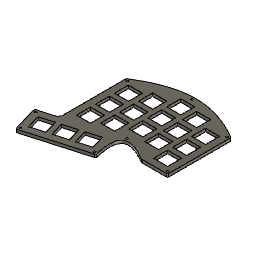
mrkabuda_switch_plate_19 v3 (Autodesk Fusion 360 design; units mm, degrees)
Autodesk Fusion 360 part; units mm, degrees
sketch "Sketch1" plane through (0, 0, 0) normal (0, 0, 1) x (1, 0, 0)
  line L0 (-65.1137, -18.4026) -> (-58.0679, -42.9099)
  line L1 (-56.8305, -43.5946) -> (3.7699, -26.1721)
  line L2 (32.056, -7.0618) -> (56.5101, -7.0618)
  line L3 (57.5101, -6.0618) -> (57.5101, 55.7146)
  line L4 (-45.9899, 54.3854) -> (-45.9899, -8.099)
  line L5 (-49.6083, -12.9043) -> (-64.4289, -17.1652)
  line L6 (-39.2399, 50.5) -> (-25.2399, 50.5)
  line L7 (-25.2399, 50.5) -> (-25.2399, 36.5)
  line L8 (-25.2399, 36.5) -> (-39.2399, 36.5)
  line L9 (-39.2399, 36.5) -> (-39.2399, 50.5)
  line L10 (-39.2399, 31.5) -> (-25.2399, 31.5)
  line L11 (-25.2399, 31.5) -> (-25.2399, 17.5)
  line L12 (-25.2399, 17.5) -> (-39.2399, 17.5)
  line L13 (-39.2399, 17.5) -> (-39.2399, 31.5)
  line L14 (-39.2399, 12.5) -> (-25.2399, 12.5)
  line L15 (-25.2399, 12.5) -> (-25.2399, -1.5)
  line L16 (-25.2399, -1.5) -> (-39.2399, -1.5)
  line L17 (-39.2399, -1.5) -> (-39.2399, 12.5)
  line L18 (-6.2399, 17.7863) -> (-6.2399, 3.7863)
  line L19 (-20.2399, 17.7863) -> (-6.2399, 17.7863)
  line L20 (-6.2399, 3.7863) -> (-20.2399, 3.7863)
  line L21 (-6.2399, 36.7863) -> (-6.2399, 22.7863)
  line L22 (-6.2399, 22.7863) -> (-20.2399, 22.7863)
  line L23 (-6.2399, 55.7863) -> (-6.2399, 41.7863)
  line L24 (-20.2399, 41.7863) -> (-20.2399, 55.7863)
  line L25 (-20.2399, 22.7863) -> (-20.2399, 36.7863)
  line L26 (-20.2399, 36.7863) -> (-6.2399, 36.7863)
  line L27 (-6.2399, 41.7863) -> (-20.2399, 41.7863)
  line L28 (-20.2399, 55.7863) -> (-6.2399, 55.7863)
  line L29 (-20.2399, 3.7863) -> (-20.2399, 17.7863)
  line L30 (12.7601, 26.8291) -> (12.7601, 12.8291)
  line L31 (-1.2399, 26.8291) -> (12.7601, 26.8291)
  line L32 (12.7601, 12.8291) -> (-1.2399, 12.8291)
  line L33 (12.7601, 45.8291) -> (12.7601, 31.8291)
  line L34 (12.7601, 31.8291) -> (-1.2399, 31.8291)
  line L35 (12.7601, 64.8291) -> (12.7601, 50.8291)
  line L36 (-1.2399, 50.8291) -> (-1.2399, 64.8291)
  line L37 (-1.2399, 31.8291) -> (-1.2399, 45.8291)
  line L38 (-1.2399, 45.8291) -> (12.7601, 45.8291)
  line L39 (12.7601, 50.8291) -> (-1.2399, 50.8291)
  line L40 (-1.2399, 64.8291) -> (12.7601, 64.8291)
  line L41 (-1.2399, 12.8291) -> (-1.2399, 26.8291)
  line L42 (31.7601, 23.77) -> (31.7601, 9.77)
  line L43 (17.7601, 23.77) -> (31.7601, 23.77)
  line L44 (31.7601, 9.77) -> (17.7601, 9.77)
  line L45 (31.7601, 42.77) -> (31.7601, 28.77)
  line L46 (31.7601, 28.77) -> (17.7601, 28.77)
  line L47 (31.7601, 61.77) -> (31.7601, 47.77)
  line L48 (17.7601, 47.77) -> (17.7601, 61.77)
  line L49 (17.7601, 28.77) -> (17.7601, 42.77)
  line L50 (17.7601, 42.77) -> (31.7601, 42.77)
  line L51 (31.7601, 47.77) -> (17.7601, 47.77)
  line L52 (17.7601, 61.77) -> (31.7601, 61.77)
  line L53 (17.7601, 9.77) -> (17.7601, 23.77)
  line L54 (50.7601, 13.6882) -> (50.7601, -0.3118)
  line L55 (36.7601, 13.6882) -> (50.7601, 13.6882)
  line L56 (50.7601, -0.3118) -> (36.7601, -0.3118)
  line L57 (50.7601, 32.6882) -> (50.7601, 18.6882)
  line L58 (50.7601, 18.6882) -> (36.7601, 18.6882)
  line L59 (50.7601, 51.6882) -> (50.7601, 37.6882)
  line L60 (36.7601, 37.6882) -> (36.7601, 51.6882)
  line L61 (36.7601, 18.6882) -> (36.7601, 32.6882)
  line L62 (36.7601, 32.6882) -> (50.7601, 32.6882)
  line L63 (50.7601, 37.6882) -> (36.7601, 37.6882)
  line L64 (36.7601, 51.6882) -> (50.7601, 51.6882)
  line L65 (36.7601, -0.3118) -> (36.7601, 13.6882)
  line L66 (-57.0377, -22.0637) -> (-53.1694, -35.5187)
  line L67 (-53.1694, -35.5187) -> (-39.7144, -31.6504)
  line L68 (-39.7144, -31.6504) -> (-43.5827, -18.1954)
  line L69 (-43.5827, -18.1954) -> (-57.0377, -22.0637)
  line L70 (-38.7774, -16.8139) -> (-34.9091, -30.2689)
  line L71 (-34.9091, -30.2689) -> (-21.4541, -26.4006)
  line L72 (-21.4541, -26.4006) -> (-25.3224, -12.9456)
  line L73 (-25.3224, -12.9456) -> (-38.7774, -16.8139)
  line L74 (-7.0621, -7.6958) -> (-20.517, -11.5641)
  line L75 (-3.1938, -21.1508) -> (-7.0621, -7.6958)
  line L76 (-20.517, -11.5641) -> (-16.6488, -25.019)
  line L77 (-16.6488, -25.019) -> (-3.1938, -21.1508)
  arc A0 (30.9232, -6.9303) -> (32.056, -7.0618) centre (32.0625, -2.0618) ccw
  arc A1 (56.5101, -7.0618) -> (57.5101, -6.0618) centre (56.5101, -6.0618) ccw
  arc A2 (-49.6083, -12.9043) -> (-45.9899, -8.099) centre (-50.9899, -8.099) ccw
  arc A3 (-64.4289, -17.1652) -> (-65.1137, -18.4026) centre (-64.1526, -18.1263) ccw
  arc A4 (-58.0679, -42.9099) -> (-56.8305, -43.5946) centre (-57.1068, -42.6336) ccw
  spline S0 degree 5 poles (4.4658, -24.9769) (4.0861, -23.4005) (3.405, -20.3536) (2.618, -16.1015) (2.0468, -11.0788) (2.1888, -5.9515) (3.2681, -2.0775) (5.3643, 0.4418) (8.517, 1.5538) (12.6793, 1.3152) (17.7712, -0.1754) (22.5239, -2.2909) (26.4446, -4.3657) (29.214, -5.9628) (30.6376, -6.8147) knots 0 0 0 0 0 0 0.1 0.2 0.3 0.4 0.5 0.6 0.7 0.8 0.9 1 1 1 1 1 1
  spline S1 degree 5 poles (-45.5293, 55.2274) (-43.5173, 56.5166) (-39.4897, 58.9843) (-33.4382, 62.3543) (-25.3488, 66.1735) (-15.1999, 69.7485) (-5.0108, 72.0184) (5.2219, 72.8785) (15.4996, 72.2738) (25.8202, 70.2648) (36.1806, 66.9583) (44.4983, 63.3605) (50.7521, 60.1603) (54.9281, 57.8074) (57.0178, 56.5761) knots 0 0 0 0 0 0 0.1 0.2 0.3 0.4 0.5 0.6 0.7 0.8 0.9 1 1 1 1 1 1
  arc A5 (57.5101, 55.7146) -> (57.0178, 56.5761) centre (56.5101, 55.7146) ccw
  arc A6 (-45.5293, 55.2274) -> (-45.9899, 54.3854) centre (-44.9899, 54.3854) ccw
  arc A7 (3.7699, -26.1721) -> (4.4658, -24.9769) centre (3.4936, -25.2111) ccw
  arc A8 (30.6376, -6.8147) -> (30.9232, -6.9303) centre (31.1511, -5.9566) ccw
  line L78 (6.3992, -33.0044) -> (2.5325, -16.9495)
  circle A9 centre (-43.4899, 53.565) radius 1.05
  line L79 (-55.3639, 48.9264) -> (-35.6948, 61.5285)
  circle A10 centre (4.9998, 70.0097) radius 1.05
  line L80 (-4.8791, 72.3551) -> (14.8791, 72.6649)
  circle A11 centre (55.0101, 54.8574) radius 1.05
  line L81 (46.894, 62.5413) -> (67.1415, 50.611)
  circle A12 centre (55.0101, -4.5618) radius 1.05
  circle A13 centre (6.2551, 3.6516) radius 1.05
  circle A14 centre (1.6991, -24.1662) radius 1.05
  line L82 (3.2764, -1.6283) -> (7.7236, 1.6283)
  circle A15 centre (-56.0797, -40.7775) radius 1.05
  circle A16 centre (-62.2965, -19.1534) radius 1.05
  point P0 (-57.7916, -43.8709)
  point P1 (5.5, 0)
  point P2 (5, 72.51)
  dimension "d1" = 27.5
  dimension "d2" = 14
  dimension "d3" = 14
  dimension "d4" = 14
  dimension "d5" = 14
  dimension "d6" = 14
  dimension "d7" = 14
  dimension "d18" = 14
  dimension "d19" = 14
  dimension "d20" = 14
  dimension "d21" = 14
  dimension "d22" = 14
  dimension "d23" = 14
  dimension "d26" = 14
  dimension "d27" = 14
  dimension "d28" = 14
  dimension "d29" = 14
  dimension "d30" = 14
  dimension "d31" = 14
  dimension "d34" = 14
  dimension "d35" = 14
  dimension "d36" = 14
  dimension "d37" = 14
  dimension "d38" = 14
  dimension "d39" = 14
  dimension "d42" = 14
  dimension "d43" = 14
  dimension "d44" = 14
  dimension "d45" = 14
  dimension "d46" = 14
  dimension "d47" = 14
  dimension "d48" = 5
  dimension "d50" = 5
  dimension "d51" = 5
  dimension "d52" = 5
  dimension "d53" = 5
  dimension "d54" = 5
  dimension "d55" = 5
  dimension "d59" = 5
  dimension "d66" = 14
  dimension "d67" = 14
  dimension "d70" = 14
  dimension "d71" = 14
  dimension "d73" = 14
  dimension "d74" = 14
  dimension "d77" = 6.75
  dimension "d80" = 1
  dimension "d83" = 5
  dimension "d85" = 1
  dimension "d86" = 1
  dimension "d135" = 6.75
  dimension "d139" = 1
  dimension "d140" = 1
  dimension "d141" = 1
  dimension "d142" = 1
  dimension "d175" = 2.1
  dimension "d176" = 2.5
  dimension "d177" = 2.5
  dimension "d178" = 2.1
  dimension "d179" = 2.5
  dimension "d180" = 2.1
  dimension "d181" = 2.5
  dimension "d182" = 2.5
  dimension "d183" = 2.1
  dimension "d184" = 2.5
  dimension "d185" = 2.5
  dimension "d186" = 2.1
  dimension "d187" = 2.1
  dimension "d188" = 2.5
  dimension "d189" = 2.5
  dimension "d190" = 2.5
  dimension "d191" = 2.1
  dimension "d192" = 2.5
  dimension "d193" = 2.5
  dimension "d194" = 2.1
  dimension "d195" = 2.5
  dimension "d196" = 2.5
  dimension "d197" = 6.75
  dimension "d198" = 6.75
  dimension "d199" = 6.75
  dimension "d201" = 5
  dimension "d202" = 6.75
  dimension "d203" = 6.75
  dimension "d204" = 5
  dimension "d205" = 5
  dimension "d206" = 5
  dimension "d207" = 5
  dimension "d208" = 5
  dimension "d209" = 5
  dimension "d210" = 5
  dimension "d211" = 5
  dimension "d212" = 5
  dimension "d214" = 5
  dimension "d215" = 5
  constraint horizontal L2
  constraint perpendicular L2 L3
  constraint perpendicular L2 L4
  constraint horizontal L6
  constraint vertical L7
  constraint horizontal L8
  constraint vertical L9
  constraint horizontal L10
  constraint vertical L11
  constraint horizontal L12
  constraint vertical L13
  constraint horizontal L14
  constraint vertical L15
  constraint horizontal L16
  constraint vertical L17
  constraint horizontal L28
  constraint vertical L23
  constraint horizontal L27
  constraint vertical L24
  constraint horizontal L26
  constraint vertical L21
  constraint horizontal L22
  constraint vertical L25
  constraint horizontal L19
  constraint vertical L18
  constraint horizontal L20
  constraint vertical L29
  constraint horizontal L40
  constraint vertical L35
  constraint horizontal L39
  constraint vertical L36
  constraint horizontal L38
  constraint vertical L33
  constraint horizontal L34
  constraint vertical L37
  constraint horizontal L31
  constraint vertical L30
  constraint horizontal L32
  constraint vertical L41
  constraint horizontal L52
  constraint vertical L47
  constraint horizontal L51
  constraint vertical L48
  constraint horizontal L50
  constraint vertical L45
  constraint horizontal L46
  constraint vertical L49
  constraint horizontal L43
  constraint vertical L42
  constraint horizontal L44
  constraint vertical L53
  constraint horizontal L64
  constraint vertical L59
  constraint horizontal L63
  constraint vertical L60
  constraint horizontal L62
  constraint vertical L57
  constraint horizontal L58
  constraint vertical L61
  constraint horizontal L55
  constraint vertical L54
  constraint horizontal L56
  constraint vertical L65
  constraint perpendicular L66 L67
  constraint parallel L66 L68
  constraint parallel L67 L69
  constraint parallel L0 L66
  constraint perpendicular L70 L71
  constraint parallel L70 L72
  constraint parallel L71 L73
  constraint parallel L68 L70
  constraint parallel L5 L69
  constraint parallel L1 L67
  constraint perpendicular L76 L77
  constraint parallel L75 L76
  constraint parallel L74 L77
  constraint collinear L73 L74
  constraint collinear L69 L73
  constraint tangent L4 A2
  constraint tangent L5 A2
  constraint tangent L0 A3
  constraint tangent L5 A3
  constraint coincident P0 L0
  constraint coincident P0 L1
  constraint tangent L0 A4
  constraint tangent L1 A4
  constraint tangent L3 A5
  constraint tangent S1 A5
  constraint tangent L4 A6
  constraint tangent S1 A6
  constraint tangent L1 A7
  constraint tangent S0 A7
  constraint tangent A0 A8
  constraint tangent S0 A8
  constraint midpoint S0.start L78
  constraint midpoint S1.start L79
  constraint midpoint P2 L80
  constraint midpoint S1.end L81
  constraint midpoint P1 L82
  constraint collinear L57 L59
  constraint collinear L54 L57
  constraint collinear L45 L47
  constraint collinear L42 L45
  measures "d2" distance of L6.start L6.end
  measures "d3" distance of L6.start L8.end
  measures "d4" distance of L10.start L12.end
  measures "d5" distance of L10.start L10.end
  measures "d6" distance of L14.start L14.end
  measures "d7" distance of L14.start L16.end
  measures "d18" distance of L24.end L23.start
  measures "d19" distance of L24.end L24.start
  measures "d20" distance of L25.end L22.end
  measures "d21" distance of L21.start L25.end
  measures "d22" distance of L18.start L19.start
  measures "d23" distance of L20.end L19.start
  measures "d26" distance of L36.end L35.start
  measures "d27" distance of L36.end L36.start
  measures "d28" distance of L37.end L34.end
  measures "d29" distance of L33.start L37.end
  measures "d30" distance of L30.start L31.start
  measures "d31" distance of L32.end L31.start
  measures "d34" distance of L48.end L47.start
  measures "d35" distance of L48.end L48.start
  measures "d36" distance of L49.end L46.end
  measures "d37" distance of L45.start L49.end
  measures "d38" distance of L42.start L43.start
  measures "d39" distance of L44.end L43.start
  measures "d42" distance of L60.end L59.start
  measures "d43" distance of L60.end L60.start
  measures "d44" distance of L61.end L58.end
  measures "d45" distance of L57.start L61.end
  measures "d46" distance of L54.start L55.start
  measures "d47" distance of L56.end L55.start
  measures "d48" distance of L62 L63
  measures "d50" distance of L7 L24
  measures "d51" distance of L11 L25
  measures "d52" distance of L15 L29
  measures "d53" distance of L23 L36
  measures "d54" distance of L21 L37
  measures "d55" distance of L18 L41
  measures "d59" distance of L47 L60
  measures "d70" distance of L70.start L70.end
  measures "d71" distance of L70.start L72.end
  measures "d74" distance of L74.end L74.start
  measures "d80" radius of A1
  measures "d83" radius of A2
  measures "d85" radius of A3
  measures "d86" radius of A4
  measures "d139" radius of A5
  measures "d140" radius of A6
  measures "d141" radius of A7
  measures "d142" radius of A8
  measures "d175" diameter of A9
  measures "d176" distance of L4 A9.centre
  measures "d177" distance of A9.centre L79
  measures "d178" diameter of A10
  measures "d179" distance of A10.centre L80
  measures "d180" diameter of A11
  measures "d181" distance of L3 A11.centre
  measures "d182" distance of A11.centre L81
  measures "d183" diameter of A12
  measures "d184" distance of L3 A12.centre
  measures "d185" distance of L2 A12.centre
  measures "d186" diameter of A13
  measures "d187" diameter of A14
  measures "d188" distance of A13.centre L82
  measures "d189" distance of L1 A14.centre
  measures "d190" distance of L78 A14.centre
  measures "d191" diameter of A15
  measures "d192" distance of L1 A15.centre
  measures "d193" distance of L0 A15.centre
  measures "d194" diameter of A16
  measures "d195" distance of L5 A16.centre
  measures "d197" distance of L4 L9
  measures "d198" distance of L4 L13
  measures "d199" distance of L4 L17
  measures "d201" distance of L55 L58
  measures "d202" distance of L2 L56
  measures "d203" distance of L3 L59
  measures "d204" distance of L35 L48
  measures "d205" distance of L50 L51
  measures "d206" distance of L43 L46
  measures "d207" distance of L31 L34
  measures "d208" distance of L38 L39
  measures "d209" distance of L26 L27
  measures "d210" distance of L19 L22
  measures "d211" distance of L8 L10
  measures "d212" distance of L12 L14
  measures "d214" distance of L68 L70
  measures "d215" distance of L72 L76
extrude "Extrude3" add sketch "Sketch1" along normal blind 3
